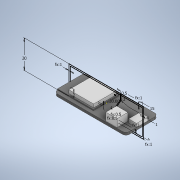
# Autodesk Inventor part: SmartEgg
Saved by Autodesk Inventor 2020 (Build 240168000, 168)
## iProperties
Created: 2019-11-26
Part Number: SmartEgg
Material: Generic
Document SubType Name: Modeling
Designer: Andrew
Density: 1 g/cm^3
Appearance: Default
Author: Andrew
Autodesk Inventor part; units mm, degrees
ref_plane "YZ Plane" through (0, 0, 0) normal (1, 0, 0) x (0, 1, 0)
ref_plane "XZ Plane" through (0, 0, 0) normal (0, 1, 0) x (-1, 0, 0)
ref_plane "XY Plane" through (0, 0, 0) normal (0, 0, 1) x (1, 0, 0)
sketch "Sketch1" plane through (0, 0, 0) normal (0, 0, 1) x (1, 0, 0)
  line L0 (-25.5, 0) -> (25.5, 0)
  line L1 (25.5, 0) -> (25.5, -1.75)
  line L2 (25.5, -1.75) -> (-25.5, -1.75)
  line L3 (-25.5, -1.75) -> (-25.5, 0)
  line L4 (0, 0) -> (-25.5, 0)
  line L5 (-25.5, 0) -> (-25.5, 0.8)
  line L6 (-25.5, 0.8) -> (0, 0.8)
  line L7 (0, 0.8) -> (0, 0)
  line L8 (-0.9, 0.8) -> (-18.55, 0.8)
  line L9 (-18.55, 0.8) -> (-18.55, 3.15)
  line L10 (-18.55, 3.15) -> (-0.9, 3.15)
  line L11 (-0.9, 3.15) -> (-0.9, 0.8)
  line L12 (10.75, 0) -> (18.75, 0)
  line L13 (18.75, 0) -> (18.75, 5.5)
  line L14 (18.75, 5.5) -> (10.75, 5.5)
  line L15 (10.75, 5.5) -> (10.75, 0)
  line L16 (25.6, 0) -> (19.95, 0)
  line L17 (19.95, 0) -> (19.95, 2.5)
  line L18 (19.95, 2.5) -> (25.6, 2.5)
  line L19 (25.6, 2.5) -> (25.6, 0)
  point P0 (0, 0)
  point P1 (0, 0)
  point P2 (19.95, 0)
  dimension "d0" = 51
  dimension "d1" = 1.75
  dimension "d2" = 0.8
  dimension "d3" = 25.5
  dimension "d4" = 17.65
  dimension "d5" = 2.35
  dimension "d6" = 24.6
  dimension "d7" = 8
  dimension "d8" = 5.5
  dimension "d9" = 14.75
  dimension "d10" = 2.5
  dimension "d11" = 5.65
  dimension "d25" = 0.1
  constraints: 40 end point, 10 parallel, 5 horizontal, 5 perpendicular, 3 point on line, 2 midpoint, 1 coincident, 1 collinear
  measures "d0" distance of L1.end L2.end
  measures "d1" distance of L0.end L1.end
  measures "d2" distance of L6.end L4.start
  measures "d3" distance of L5.end L6.end
  measures "d4" distance of L9.end L10.end
  measures "d5" distance of L10.end L8.start
  measures "d6" distance between parallel lines of L5 L11
  measures "d7" distance of L13.end L14.end
  measures "d8" distance of L12.end L13.end
  measures "d9" distance between parallel lines of L1 L15
  measures "d10" distance of L16.start L18.end
  measures "d11" distance of L17.end L18.end
  measures "d25" distance between parallel lines of L1 L19
extrude "PCB" add sketch "Sketch1" along normal mid plane 22.85 contours L0 L1 L2 L3
fillet "Fillet1" radius 2.5 4 edges at (-25.5, -0.875, 11.425) (-25.5, -0.875, -11.425) (25.5, -0.875, -11.425) (25.5, -0.875, 11.425)
extrude "ESP32PCB" add sketch "Sketch1" along normal mid plane 18.1 contours L5 L6 L7 L0
extrude "ESP32Shied" add sketch "Sketch1" along normal mid plane 15.9 contours L9 L10 L11 L6
extrude "Battery Connector" add sketch "Sketch1" along normal blind 11 contours L15 L14 L13 L0
extrude "Extrusion5" cut sketch "Sketch1" along normal blind 3.3 contours L15 L14 L13 L0
extrude "Extrusion6" add sketch "Sketch1" along normal mid plane 8 contours L0 L17 L18 L19 L16
sketch "Sketch2" plane through (0, 0, 0) normal (0, 0, 1) x (1, 0, 0)
  line L0 (25.5, 10.25) -> (25.5, -7.75)
  line L1 (26.5, 11.25) -> (26.5, -8.75)
  line L2 (-26.5, -8.75) -> (-26.5, 11.25)
  line L3 (25.5, 0) -> (25.5, -1.75) construction
  line L4 (-25.5, -1.75) -> (-25.5, 0) construction
  line L5 (-25.5, 0) -> (-25.5, -1.75) projected
  line L6 (-25.5, -1.75) -> (-5.7719, -1.75)
  line L7 (-5.7719, -1.75) -> (-5.7719, -2.75)
  line L8 (-5.7719, -2.75) -> (-25.5, -2.75)
  line L9 (-25.5, -7.75) -> (-25.5, -2.75)
  line L10 (-25.5, -1.75) -> (-25.5, 10.25)
  line L11 (10.5, 11.25) -> (10.5, 10.25)
  line L12 (10, 11.25) -> (10, 10.25)
  line L13 (3.6547, -7.75) -> (3.6547, -8.75)
  line L14 (3.1547, -8.75) -> (3.1547, -7.75)
  line L15 (25.5, -7.75) -> (3.6547, -7.75)
  line L16 (3.1547, -7.75) -> (-25.5, -7.75)
  line L17 (26.5, -8.75) -> (3.6547, -8.75)
  line L18 (3.1547, -8.75) -> (-26.5, -8.75)
  line L19 (-25.5, 10.25) -> (10, 10.25)
  line L20 (10.5, 10.25) -> (25.5, 10.25)
  line L21 (-26.5, 11.25) -> (10, 11.25)
  line L22 (10.5, 11.25) -> (26.5, 11.25)
  line L23 (9.9641, 6.25) -> (4.1906, -3.75)
  line L24 (3.6547, -5.75) -> (3.6547, -7.75)
  line L25 (10.5, 8.25) -> (10.5, 10.25)
  line L26 (10, 10.25) -> (10, 8.384)
  line L27 (9.4641, 6.384) -> (3.6906, -3.616)
  line L28 (3.1547, -5.616) -> (3.1547, -7.75)
  arc A0 (9.4641, 6.384) -> (10, 8.384) centre (6, 8.384) ccw
  arc A1 (9.9641, 6.25) -> (10.5, 8.25) centre (6.5, 8.25) ccw
  arc A2 (3.6906, -3.616) -> (3.1547, -5.616) centre (7.1547, -5.616) ccw
  arc A3 (4.1906, -3.75) -> (3.6547, -5.75) centre (7.6547, -5.75) ccw
  point P0 (0, 0)
  point P1 (-10.486, 0)
  dimension "d27" = 1
  dimension "d30" = 1
  dimension "d31" = 5
  dimension "d32" = 1
  dimension "d34" = 1
  dimension "d35" = 1
  dimension "d36" = 0.5
  dimension "d37" = 0.5
  dimension "d39" = 30
  dimension "d40" = 0.5
  dimension "d41" = 4
  dimension "d42" = 2
  dimension "d43" = 2
  dimension "d44" = 20
  dimension "d46" = 15
  constraints: 52 end point, 17 parallel, 9 perpendicular, 8 point on circle, 8 tangent, 7 collinear, 5 horizontal, 4 centre point, 3 equal radius, 2 vertical
  measures "d27" distance between parallel lines of L1 L0
  measures "d30" distance of L6.end L7.end
  measures "d31" distance of L9.start L8.end
  measures "d32" distance between parallel lines of L20 L22
  measures "d34" distance between parallel lines of L17 L15
  measures "d35" distance between parallel lines of L2 L10
  measures "d36" distance between parallel lines of L11 L12
  measures "d37" distance between parallel lines of L23 L27
  measures "d39" angle of L24 L23
  measures "d40" distance between parallel lines of L28 L24
  measures "d41" radius of A0
  measures "d42" distance of L25.start L11.end
  measures "d43" distance of L24.start L13.start
  measures "d44" distance between parallel lines of L18 L21
  measures "d46" distance between parallel lines of L0 L25
equation "\"d32\" = d27"
equation "\"d34\" = d27"
equation "\"d35\" = d27"
equation "\"d37\" = d36"
equation "\"d40\" = d36"
equation "\"d43\" = d42"
equation "\"d28\" = d26"
equation "\"d29\" = d26"
equation "\"d26\" = 1"
body "Solid1"
